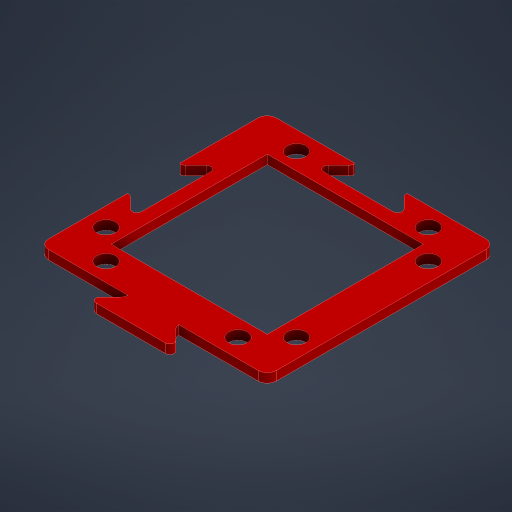
# Autodesk Inventor part: Interlinking Baseplate Edge V4
Saved by Autodesk Inventor 2023.4 (Build 274418000, 418)
## iProperties
Created: 2024-07-23
Part Number: Interlinking Baseplate Edge V4
Material: Generic
Document SubType Name: Modeling
Designer: xSibe
Density: 1 g/cm^3
Appearance: Plastic Dark Red
Author: xSibe
Autodesk Inventor part; units mm, degrees
ref_plane "YZ Plane" through (0, 0, 0) normal (1, 0, 0) x (0, 1, 0)
ref_plane "XZ Plane" through (0, 0, 0) normal (0, 1, 0) x (-1, 0, 0)
ref_plane "XY Plane" through (0, 0, 0) normal (0, 0, 1) x (1, 0, 0)
sketch "Sketch1" plane through (0, 0, 0) normal (0, 1, 0) x (-1, 0, 0)
  circle A0 centre (-21.9, -21.9) radius 1.875 projected
  circle A1 centre (21.9, 21.9) radius 1.875 projected
  circle A2 centre (21.9, -21.9) radius 1.875 projected
  circle A3 centre (-21.9, 21.9) radius 1.875 projected
  circle A4 centre (14.4, 20.8) radius 2.0734 projected
  circle A5 centre (-14.4, -20.8) radius 2.0734 projected
  circle A6 centre (14.4, -20.8) radius 2.0734 projected
  circle A7 centre (20.8, -14.4) radius 2.0734 projected
  line L0 (-17.05, 17.05) -> (-17.05, -17.05) projected
  line L1 (17.05, 17.05) -> (-17.05, 17.05) projected
  line L2 (17.05, -17.05) -> (17.05, 17.05) projected
  line L3 (-17.05, -17.05) -> (17.05, -17.05) projected
  circle A8 centre (20.8, 14.4) radius 2.0734 projected
  circle A9 centre (-14.4, 20.8) radius 2.0734 projected
  circle A10 centre (-20.8, -14.4) radius 2.0734 projected
  circle A11 centre (-20.8, 14.4) radius 2.0734 projected
  line L4 (-22.9, 24.875) -> (22.9, 24.875) projected
  arc A12 (-22.9, 24.875) -> (-24.875, 22.9) centre (-22.9, 22.9) ccw projected
  line L5 (-24.875, -22.9) -> (-24.875, 22.9) projected
  arc A13 (-24.875, -22.9) -> (-22.9, -24.875) centre (-22.9, -22.9) ccw projected
  line L6 (22.9, -24.875) -> (-22.9, -24.875) projected
  arc A14 (22.9, -24.875) -> (24.875, -22.9) centre (22.9, -22.9) ccw projected
  line L7 (24.875, 22.9) -> (24.875, -22.9) projected
  arc A15 (24.875, 22.9) -> (22.9, 24.875) centre (22.9, 22.9) ccw projected
  arc A16 (24.9, 22.9) -> (22.9, 24.9) centre (22.9, 22.9) ccw projected
  line L8 (22.9, 24.9) -> (-22.9, 24.9) projected
  arc A17 (-22.9, 24.9) -> (-24.9, 22.9) centre (-22.9, 22.9) ccw projected
  line L9 (-24.9, 22.9) -> (-24.9, -22.9) projected
  arc A18 (-24.9, -22.9) -> (-22.9, -24.9) centre (-22.9, -22.9) ccw projected
  line L10 (-22.9, -24.9) -> (22.9, -24.9) projected
  arc A19 (22.9, -24.9) -> (24.9, -22.9) centre (22.9, -22.9) ccw projected
  line L11 (24.9, -22.9) -> (24.9, 22.9) projected
  point P0 (0, 0)
extrude "Extrusion1" add sketch "Sketch1" along normal blind 2 contours A0 | A1 | A2 | A3 | A7 | L4 A15 L7 A14 L6 A13 L5 A12
sketch "Sketch2" plane through (0, 0, 0) normal (0, 1, 0) x (-1, 0, 0)
  line L0 (-22.9, -24.875) -> (22.9, -24.875) projected
  arc A0 (22.9, -24.875) -> (24.875, -22.9) centre (22.9, -22.9) ccw projected
  line L1 (24.875, -22.9) -> (24.875, 22.9) projected
  arc A1 (24.875, 22.9) -> (22.9, 24.875) centre (22.9, 22.9) ccw projected
  line L2 (22.9, 24.875) -> (-22.9, 24.875) projected
  arc A2 (-22.9, 24.875) -> (-24.875, 22.9) centre (-22.9, 22.9) ccw projected
  line L3 (-24.875, 22.9) -> (-24.875, -22.9) projected
  arc A3 (-24.875, -22.9) -> (-22.9, -24.875) centre (-22.9, -22.9) ccw projected
  circle A4 centre (-20.8, 14.4) radius 2.0734 projected
  circle A5 centre (-20.8, -14.4) radius 2.0734 projected
  circle A6 centre (-14.4, 20.8) radius 2.0734 projected
  circle A7 centre (20.8, 14.4) radius 2.0734 projected
  circle A8 centre (14.4, -20.8) radius 2.0734 projected
  circle A9 centre (-14.4, -20.8) radius 2.0734 projected
  circle A10 centre (14.4, 20.8) radius 2.0734 projected
  line L4 (-17.05, 17.05) -> (17.05, 17.05) projected
  line L5 (17.05, 17.05) -> (17.05, -17.05) projected
  line L6 (17.05, -17.05) -> (-17.05, -17.05) projected
  line L7 (-17.05, -17.05) -> (-17.05, 17.05) projected
  line L8 (-7.5858, 19.875) -> (7.5858, 19.875)
  line L9 (10, 19.875) -> (10, 29.875)
  line L10 (7.5858, 29.875) -> (-7.5858, 29.875)
  line L11 (-10, 29.875) -> (-10, 19.875)
  line L12 (-10, 19.875) -> (10, 29.875) construction
  line L13 (10, 19.875) -> (-10, 29.875) construction
  line L14 (-8.2929, 28.1679) -> (-6.0607, 25.9357)
  line L15 (-10, 29.875) -> (-6.8431, 29.875) construction
  line L16 (8.2929, 28.1679) -> (6.0607, 25.9357)
  line L17 (10, 29.875) -> (13.1569, 29.875) construction
  line L18 (5, 24.875) -> (-5, 24.875)
  line L19 (-8.2929, 21.5821) -> (-6.0607, 23.8143)
  line L20 (8.2929, 21.5821) -> (6.0607, 23.8143)
  arc A11 (-8.2929, 21.5821) -> (-7.5858, 19.875) centre (-7.5858, 20.875) ccw
  arc A12 (7.5858, 19.875) -> (8.2929, 21.5821) centre (7.5858, 20.875) ccw
  arc A13 (-6.0607, 23.8143) -> (-6.0607, 25.9357) centre (-7.1213, 24.875) ccw
  arc A14 (6.0607, 25.9357) -> (6.0607, 23.8143) centre (7.1213, 24.875) ccw
  arc A15 (-7.5858, 29.875) -> (-8.2929, 28.1679) centre (-7.5858, 28.875) ccw
  arc A16 (8.2929, 28.1679) -> (7.5858, 29.875) centre (7.5858, 28.875) ccw
  line L21 (-7.5858, 29.8) -> (7.5858, 29.8)
  arc A17 (8.2399, 28.2209) -> (7.5858, 29.8) centre (7.5858, 28.875) ccw
  line L22 (8.2399, 28.2209) -> (6.0076, 25.9887)
  arc A18 (6.0076, 25.9887) -> (6.0076, 23.7613) centre (7.1213, 24.875) ccw
  line L23 (6.0076, 23.7613) -> (8.2399, 21.5291)
  arc A19 (7.5858, 19.95) -> (8.2399, 21.5291) centre (7.5858, 20.875) ccw
  line L24 (7.5858, 19.95) -> (-7.5858, 19.95)
  arc A20 (-8.2399, 21.5291) -> (-7.5858, 19.95) centre (-7.5858, 20.875) ccw
  line L25 (-8.2399, 21.5291) -> (-6.0076, 23.7613)
  arc A21 (-6.0076, 23.7613) -> (-6.0076, 25.9887) centre (-7.1213, 24.875) ccw
  line L26 (-6.0076, 25.9887) -> (-8.2399, 28.2209)
  arc A22 (-7.5858, 29.8) -> (-8.2399, 28.2209) centre (-7.5858, 28.875) ccw
  arc A23 (-21.5291, -8.2399) -> (-19.95, -7.5858) centre (-20.875, -7.5858) ccw
  arc A24 (-21.5821, -8.2929) -> (-19.875, -7.5858) centre (-20.875, -7.5858) ccw
  line L27 (-25.9887, -6.0076) -> (-28.2209, -8.2399)
  line L28 (-21.5291, -8.2399) -> (-23.7613, -6.0076)
  line L29 (-21.5821, -8.2929) -> (-23.8143, -6.0607)
  arc A25 (-23.8143, -6.0607) -> (-25.9357, -6.0607) centre (-24.875, -7.1213) ccw
  arc A26 (-23.7613, -6.0076) -> (-25.9887, -6.0076) centre (-24.875, -7.1213) ccw
  line L30 (-28.1679, -8.2929) -> (-25.9357, -6.0607)
  line L31 (-24.875, 5) -> (-24.875, -5)
  line L32 (-19.95, 7.5858) -> (-19.95, -7.5858)
  line L33 (-19.875, -7.5858) -> (-19.875, 7.5858)
  line L34 (-29.8, -7.5858) -> (-29.8, 7.5858)
  line L35 (-29.875, 7.5858) -> (-29.875, -7.5858)
  arc A27 (-29.875, -7.5858) -> (-28.1679, -8.2929) centre (-28.875, -7.5858) ccw
  line L36 (-28.1679, 8.2929) -> (-25.9357, 6.0607)
  line L37 (-21.5821, 8.2929) -> (-23.8143, 6.0607)
  arc A28 (-19.875, 7.5858) -> (-21.5821, 8.2929) centre (-20.875, 7.5858) ccw
  arc A29 (-25.9887, 6.0076) -> (-23.7613, 6.0076) centre (-24.875, 7.1213) ccw
  arc A30 (-25.9357, 6.0607) -> (-23.8143, 6.0607) centre (-24.875, 7.1213) ccw
  arc A31 (-19.95, 7.5858) -> (-21.5291, 8.2399) centre (-20.875, 7.5858) ccw
  line L38 (-23.7613, 6.0076) -> (-21.5291, 8.2399)
  line L39 (-28.2209, 8.2399) -> (-25.9887, 6.0076)
  arc A32 (-28.2209, 8.2399) -> (-29.8, 7.5858) centre (-28.875, 7.5858) ccw
  arc A33 (-28.1679, 8.2929) -> (-29.875, 7.5858) centre (-28.875, 7.5858) ccw
  arc A34 (-29.8, -7.5858) -> (-28.2209, -8.2399) centre (-28.875, -7.5858) ccw
  arc A35 (8.2399, -21.5291) -> (7.5858, -19.95) centre (7.5858, -20.875) ccw
  arc A36 (8.2929, -21.5821) -> (7.5858, -19.875) centre (7.5858, -20.875) ccw
  line L40 (6.0076, -25.9887) -> (8.2399, -28.2209)
  line L41 (8.2399, -21.5291) -> (6.0076, -23.7613)
  line L42 (8.2929, -21.5821) -> (6.0607, -23.8143)
  arc A37 (6.0607, -23.8143) -> (6.0607, -25.9357) centre (7.1213, -24.875) ccw
  arc A38 (6.0076, -23.7613) -> (6.0076, -25.9887) centre (7.1213, -24.875) ccw
  line L43 (8.2929, -28.1679) -> (6.0607, -25.9357)
  line L44 (-5, -24.875) -> (5, -24.875)
  line L45 (-7.5858, -19.95) -> (7.5858, -19.95)
  line L46 (7.5858, -19.875) -> (-7.5858, -19.875)
  line L47 (7.5858, -29.8) -> (-7.5858, -29.8)
  line L48 (-7.5858, -29.875) -> (7.5858, -29.875)
  arc A39 (7.5858, -29.875) -> (8.2929, -28.1679) centre (7.5858, -28.875) ccw
  line L49 (-8.2929, -28.1679) -> (-6.0607, -25.9357)
  line L50 (-8.2929, -21.5821) -> (-6.0607, -23.8143)
  arc A40 (-7.5858, -19.875) -> (-8.2929, -21.5821) centre (-7.5858, -20.875) ccw
  arc A41 (-6.0076, -25.9887) -> (-6.0076, -23.7613) centre (-7.1213, -24.875) ccw
  arc A42 (-6.0607, -25.9357) -> (-6.0607, -23.8143) centre (-7.1213, -24.875) ccw
  arc A43 (-7.5858, -19.95) -> (-8.2399, -21.5291) centre (-7.5858, -20.875) ccw
  line L51 (-6.0076, -23.7613) -> (-8.2399, -21.5291)
  line L52 (-8.2399, -28.2209) -> (-6.0076, -25.9887)
  arc A44 (-8.2399, -28.2209) -> (-7.5858, -29.8) centre (-7.5858, -28.875) ccw
  arc A45 (-8.2929, -28.1679) -> (-7.5858, -29.875) centre (-7.5858, -28.875) ccw
  arc A46 (7.5858, -29.8) -> (8.2399, -28.2209) centre (7.5858, -28.875) ccw
  arc A47 (21.5291, 8.2399) -> (19.95, 7.5858) centre (20.875, 7.5858) ccw
  arc A48 (21.5821, 8.2929) -> (19.875, 7.5858) centre (20.875, 7.5858) ccw
  line L53 (25.9887, 6.0076) -> (28.2209, 8.2399)
  line L54 (21.5291, 8.2399) -> (23.7613, 6.0076)
  line L55 (21.5821, 8.2929) -> (23.8143, 6.0607)
  arc A49 (23.8143, 6.0607) -> (25.9357, 6.0607) centre (24.875, 7.1213) ccw
  arc A50 (23.7613, 6.0076) -> (25.9887, 6.0076) centre (24.875, 7.1213) ccw
  line L56 (28.1679, 8.2929) -> (25.9357, 6.0607)
  line L57 (24.875, -5) -> (24.875, 5)
  line L58 (19.95, -7.5858) -> (19.95, 7.5858)
  line L59 (19.875, 7.5858) -> (19.875, -7.5858)
  line L60 (29.8, 7.5858) -> (29.8, -7.5858)
  line L61 (29.875, -7.5858) -> (29.875, 7.5858)
  arc A51 (29.875, 7.5858) -> (28.1679, 8.2929) centre (28.875, 7.5858) ccw
  line L62 (28.1679, -8.2929) -> (25.9357, -6.0607)
  line L63 (21.5821, -8.2929) -> (23.8143, -6.0607)
  arc A52 (19.875, -7.5858) -> (21.5821, -8.2929) centre (20.875, -7.5858) ccw
  arc A53 (25.9887, -6.0076) -> (23.7613, -6.0076) centre (24.875, -7.1213) ccw
  arc A54 (25.9357, -6.0607) -> (23.8143, -6.0607) centre (24.875, -7.1213) ccw
  arc A55 (19.95, -7.5858) -> (21.5291, -8.2399) centre (20.875, -7.5858) ccw
  line L64 (23.7613, -6.0076) -> (21.5291, -8.2399)
  line L65 (28.2209, -8.2399) -> (25.9887, -6.0076)
  arc A56 (28.2209, -8.2399) -> (29.8, -7.5858) centre (28.875, -7.5858) ccw
  arc A57 (28.1679, -8.2929) -> (29.875, -7.5858) centre (28.875, -7.5858) ccw
  arc A58 (29.8, 7.5858) -> (28.2209, 8.2399) centre (28.875, 7.5858) ccw
  point P0 (0, 0)
  point P1 (0, 24.875)
  point P2 (-29.875, -6.8431)
  point P3 (-19.875, -10)
  point P4 (-29.875, -10)
  point P5 (-24.875, 0)
  point P6 (-19.875, 10)
  point P7 (-29.875, 10)
  point P8 (6.8431, -29.875)
  point P9 (10, -19.875)
  point P10 (10, -29.875)
  point P11 (0, -24.875)
  point P12 (-10, -19.875)
  point P13 (-10, -29.875)
  point P14 (29.875, 6.8431)
  point P15 (19.875, 10)
  point P16 (29.875, 10)
  point P17 (24.875, 0)
  point P18 (19.875, -10)
  point P19 (29.875, -10)
  point P20 (-24.875, -5.5463)
  point P21 (-24.875, 5.5463)
  point P22 (-5.5463, 24.875)
  point P23 (5.5463, 24.875)
  point P24 (5.6213, -24.875)
  point P25 (-5.6213, -24.875)
  point P26 (24.875, 5.6213)
  point P27 (24.875, -5.6213)
  dimension "d2" = 20
  dimension "d3" = 10
  dimension "d4" = 45
  dimension "d5" = 135
  dimension "d6" = 1
  dimension "d7" = 1.5
  dimension "d8" = 1
  dimension "d9" = 0.075
  dimension "d12" = 360
  constraints: 116 end point, 96 point on circle, 50 point on line, 48 centre point, 12 tangent, 3 equal radius, 3 horizontal, 3 midpoint, 3 parallel, 2 equal length, 1 collinear, 1 perpendicular, 264 other
  measures "d2" distance of L11.start L9.end
  measures "d3" distance of L9.start L9.end
  measures "d4" angle of L14 L15
  measures "d5" angle of L16 L17
  measures "d6" radius of A11
  measures "d7" radius of A13
  measures "d8" radius of A15
  measures "d9" distance between parallel lines of L10 L21
extrude "Extrusion2" add sketch "Sketch2" along normal up to surface (2 mm away) contours A21 L26 A22 L21 A17 L22 A18 L2
extrude "Extrusion3" cut sketch "Sketch2" along normal up to surface (2 mm away) contours L0 A41 L51 A43 L45 A35 L41 A38 | L0 A42 L50 A40 L46 A36 L42 A37 A38 L41 A35 L45 A43 L51 A41 | A54 L63 A52 L59 A48 L55 A49 L1 A50 L54 A47 L58 A55 L64 A53 | A53 L64 A55 L58 A47 L54 A50 L1
fillet "Fillet1" radius 0.25 4 edges at (-24.875, 1, 5.6213) (-24.875, 1, -5.6213) (5.6213, 1, -24.875) (-5.6213, 1, -24.875)
body "Solid1"
